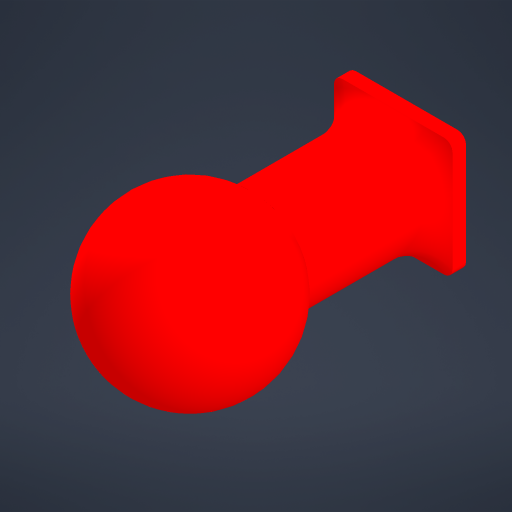
# Autodesk Inventor part: Cube Press Top
Saved by Autodesk Inventor 2023.4 (Build 274418000, 418)
## iProperties
Created: 2022-08-17
Part Number: Cube Press Top
Material: Generic
Document SubType Name: Modeling
Designer: xSibe
Density: 1 g/cm^3
Appearance: Plastic Red
Author: xSibe
Autodesk Inventor part; units mm, degrees
ref_plane "YZ Plane" through (0, 0, 0) normal (1, 0, 0) x (0, 1, 0)
sketch "Sketch1" plane through (0, 0, 0) normal (0, 0, 1) x (1, 0, 0)
  circle A0 centre (-96.7, -21.9) radius 1.875 projected
  circle A1 centre (-52.9, 21.9) radius 1.875 projected
  circle A2 centre (-52.9, -21.9) radius 1.875 projected
  circle A3 centre (-96.7, 21.9) radius 1.875 projected
  circle A4 centre (-89.2, -20.8) radius 2.0734 projected
  circle A5 centre (-60.4, -20.8) radius 2.0734 projected
  circle A6 centre (-54, -14.4) radius 2.0734 projected
  circle A7 centre (-95.6, -14.4) radius 2.0734 projected
  circle A8 centre (-95.6, 14.4) radius 2.0734 projected
  circle A9 centre (-54, 14.4) radius 2.0734 projected
  circle A10 centre (-60.4, 20.8) radius 2.0734 projected
  circle A11 centre (-89.2, 20.8) radius 2.0734 projected
  line L0 (-97.7, 24.875) -> (-51.9, 24.875) projected
  arc A12 (-97.7, 24.875) -> (-99.675, 22.9) centre (-97.7, 22.9) ccw projected
  line L1 (-99.675, -22.9) -> (-99.675, 22.9) projected
  arc A13 (-99.675, -22.9) -> (-97.7, -24.875) centre (-97.7, -22.9) ccw projected
  line L2 (-51.9, -24.875) -> (-97.7, -24.875) projected
  arc A14 (-51.9, -24.875) -> (-49.925, -22.9) centre (-51.9, -22.9) ccw projected
  line L3 (-49.925, 22.9) -> (-49.925, -22.9) projected
  arc A15 (-49.925, 22.9) -> (-51.9, 24.875) centre (-51.9, 22.9) ccw projected
  line L4 (-49.8, 25) -> (-99.8, 25)
  line L5 (-99.8, 25) -> (-99.8, -25)
  line L6 (-99.8, -25) -> (-49.8, -25)
  line L7 (-49.8, -25) -> (-49.8, 25)
  line L8 (-49.8, 25) -> (-99.8, -25) construction
  line L9 (-99.8, 25) -> (-49.8, -25) construction
  line L10 (-32.3, -7.5) -> (-67.3, -7.5)
  line L11 (-67.3, -7.5) -> (-67.3, -42.5)
  line L12 (-67.3, -42.5) -> (-32.3, -42.5)
  line L13 (-32.3, -42.5) -> (-32.3, -7.5)
  line L14 (-32.3, -7.5) -> (-67.3, -42.5) construction
  line L15 (-67.3, -7.5) -> (-32.3, -42.5) construction
  line L16 (-49.925, 0) -> (-99.675, 0)
  circle A16 centre (-54, -14.4) radius 2.0734
  circle A17 centre (-60.4, -20.8) radius 2.0734
  circle A18 centre (-60.4, -29.2) radius 2.0734
  circle A19 centre (-54, -35.6) radius 2.0734
  circle A20 centre (-45.6, -35.6) radius 2.0734
  circle A21 centre (-39.2, -29.2) radius 2.0734
  circle A22 centre (-39.2, -20.8) radius 2.0734
  circle A23 centre (-45.6, -14.4) radius 2.0734
  point P0 (-74.8, 0)
  dimension "d20" = 50
  dimension "d21" = 50
  dimension "d22" = 35
  dimension "d23" = 35
  dimension "d26" = 360
  constraints: 26 end point, 8 centre point, 7 midpoint, 4 parallel, 2 coincident, 2 concentric, 2 horizontal, 2 perpendicular, 17 other
  measures "d20" distance of L6.end L5.end
  measures "d21" distance of L5.end L4.end
  measures "d22" distance of L12.end L11.end
  measures "d23" distance of L11.end L10.end
ref_plane "Work Plane1" through (-24.875, -24.875, 49.8) normal (0, 0, 1) x (1, 0, 0)
extrude "Extrusion1" add sketch "Sketch1" along normal blind 1.5 from surface at 49.8 contours A2 | L10 L7 L6 L11 L2 A14 L3 | L3 A14 L2 L11 L10 | L10 L13 L12 L11 L6 L7
sketch "Sketch2" plane through (7.5, -7.5, 51.3) normal (0, 0, 1) x (1, 0, 0)
  line L0 (-74.8, 0) -> (-39.8, 0) projected
  line L1 (-74.8, -35) -> (-74.8, 0) projected
  line L2 (-39.8, -35) -> (-74.8, -35) projected
  line L3 (-39.8, 0) -> (-39.8, -35) projected
  circle A0 centre (-46.7, -13.3) radius 2.0734 projected
  circle A1 centre (-53.1, -28.1) radius 2.0734 projected
  circle A2 centre (-67.9, -21.7) radius 2.0734 projected
  circle A3 centre (-61.5, -28.1) radius 2.0734 projected
  circle A4 centre (-46.7, -21.7) radius 2.0734 projected
  circle A5 centre (-53.1, -6.9) radius 2.0734 projected
  circle A6 centre (-67.9, -13.3) radius 2.0734 projected
  circle A7 centre (-61.5, -6.9) radius 2.0734 projected
extrude "Extrusion2" add sketch "Sketch2" along normal blind 2.5 contours L0 L3 L2 L1 | A0 | A1 | A2 | A3 | A4 | A5 | A6 | A7
fillet "Fillet1" radius 2.5 4 edges at (-32.3, -7.5, 51.8) (-67.3, -7.5, 51.8) (-67.3, -42.5, 51.8) (-32.3, -42.5, 51.8)
sketch "Sketch3" plane through (7.5, -7.5, 53.8) normal (0, 0, 1) x (1, 0, 0)
  line L0 (-39.8, -17.5) -> (-74.8, -17.5)
  circle A0 centre (-57.3, -17.5) radius 15
  line L1 (-39.8, -32.5) -> (-39.8, -2.5) projected
  line L2 (-74.8, -2.5) -> (-74.8, -32.5) projected
  point P0 (-7.5, 7.5)
  dimension "d13" = 30
  constraints: 3 midpoint, 2 end point, 1 centre point
  measures "d13" diameter of A0
extrude "Extrusion3" add sketch "Sketch3" along normal blind 75
fillet "Fillet2" radius 15 1 edges at (-64.8, -25, 128.8)
ref_plane "Work Plane2" through (-64.8, -25, 53.8) normal (0, 1, 0) x (1, 0, 0)
sketch "Sketch4" plane through (-64.8, -25, 53.8) normal (0, 1, 0) x (1, 0, 0)
  arc A0 (0, -60) -> (30, -60) centre (15, -60) ccw projected
  circle A1 centre (15, -60) radius 25
  line L0 (15, -60) -> (15, -10)
  line L1 (15, -60) -> (15, -85)
  point P0 (64.8, 53.8)
  point P1 (15, -35)
  dimension "d17" = 50
  dimension "d18" = 50
  constraints: 4 end point, 2 vertical, 1 coincident, 3 other
  measures "d18" distance of L0.start L0.end
revolve "Revolution1" add sketch "Sketch4" angle 360 about axis through (-49.8, -25, 113.8) along (0, 0, 1) picked at (8.1418, -69.7339) contours A1 L0 L1
fillet "Fillet3" radius 10 1 edges at (-64.8, -25, 53.8)
body "Solid1"
